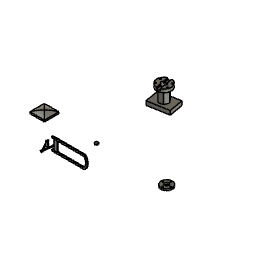
HW 1 (Autodesk Fusion 360 design; units mm, degrees)
Autodesk Fusion 360 part; units mm, degrees
note: some values were not read from the file. Set by a fixed rule: which sketch regions a step uses.
(part 1 of 2)
sketch "Sketch1" plane through (0, 0, 0) normal (0, 0, 1) x (1, 0, 0)
  line L0 (40, 0) -> (-50, 0)
  line L1 (-50, 0) -> (-50, 10)
  line L2 (-50, 10) -> (40, 10)
  line L3 (40, 10) -> (40, 0)
  line L4 (-5, 10) -> (-5, 20)
  arc A0 (40, 10) -> (-50, 10) centre (-5, -86.2) ccw
  point P0 (-5, 10)
  dimension "d1" = 10
  dimension "d2" = 90
  constraint horizontal L0
  constraint vertical L1
  constraint horizontal L2
  constraint vertical L3
  constraint midpoint L2 P0
  constraint coincident P0 L4.start
  constraint perpendicular L2 L4
  measures "d1" distance of L0.start L2.end
  measures "d2" distance of L1.end L2.end
extrude "Extrude1" add sketch "Sketch1" along normal blind 90 makes body 1
ref_plane "WorkPlane2" through (40, 5, 45) normal (1, 0, 0) x (0, 1, 0)
sketch "Sketch4" plane through (40, 5, 45) normal (1, 0, 0) x (0, 1, 0)
  line L0 (-5, 45) -> (5, 45)
  line L1 (5, 45) -> (5, -45)
  line L2 (5, -45) -> (-5, -45)
  line L3 (-5, -45) -> (-5, 45)
  line L4 (5, 0) -> (15, 0)
  arc A0 (5, -45) -> (5, 45) centre (-91.25, 0) ccw
  constraint horizontal L0
  constraint vertical L1
  constraint horizontal L2
  constraint vertical L3
  constraint midpoint L1 L4.start
  constraint perpendicular L1 L4
  constraint coincident L4.end A0
extrude "Extrude3" cut sketch "Sketch4" against normal up to surface (90 mm away) keep common part bodies 1
sketch "Sketch5" plane through (0, 0, 0) normal (0, 1, 0) x (1, 0, 0)
  circle A0 centre (220, -140) radius 35
  circle A1 centre (220, -140) radius 14
  circle A2 centre (220, -140) radius 16.5
  circle A3 centre (220, -140) radius 21
  dimension "d19" = 70
  dimension "d20" = 28
  dimension "d21" = 33
  dimension "d22" = 42
  constraint concentric A0 A1
  constraint concentric A0 A2
  constraint concentric A0 A3
  measures "d19" diameter of A0
  measures "d20" diameter of A1
  measures "d21" diameter of A2
  measures "d22" diameter of A3
extrude "Extrude4" add sketch "Sketch5" along normal blind 10 separate body contours A0 makes body 2
extrude "Extrude5" add sketch "Sketch5" along normal blind 15 contours A3 bodies 2
extrude "Extrude6" add sketch "Sketch5" along normal blind 10 contours A2 bodies 2
sketch "Sketch6" plane through (0, 10, 0) normal (0, 1, 0) x (-1, 0, 0)
  circle A0 centre (-220, 140) radius 21
  circle A1 centre (-220, 140) radius 35
ref_plane "WorkPlane3" through (220, 10, 140) normal (0, 1, 0) x (-1, 0, 0)
sketch "Sketch7" plane through (220, 10, 140) normal (0, 1, 0) x (1, 0, 0)
  circle A0 centre (0, 0) radius 25 construction
  line L0 (0, 25) -> (0, -25)
  circle A1 centre (0, -25) radius 4
  circle A2 centre (25, 0) radius 4
  circle A3 centre (0, 25) radius 4
  circle A4 centre (-25, 0) radius 4
  dimension "d30" = 50
  dimension "d31" = 8
  dimension "d33" = 360
  constraint coincident A0.centre origin
  constraint coincident A0 L0.start
  constraint coincident A0 L0.end
  constraint vertical L0
  constraint coincident L0.end A1.centre
  measures "d30" diameter of A0
  measures "d31" diameter of A1
sketch "Sketch8" plane through (220, 10, 140) normal (0, 1, 0) x (-1, 0, 0)
extrude "Extrude7" cut sketch "Sketch7" against normal up to surface (10 mm away) bodies 2
sketch "Sketch9" plane through (0, 0, 0) normal (0, 1, 0) x (1, 0, 0)
ref_plane "WorkPlane4" through (302.5, 0, -250) normal (0, -1, 0) x (1, 0, 0)
sketch "Sketch10" plane through (300, 0, -250) normal (0, -1, 0) x (1, 0, 0)
ref_plane "WorkPlane5" through (200.7071, 0, -200) normal (0, -1, 0) x (1, 0, 0)
sketch "Sketch11" plane through (230.8314, 0, -200) normal (0, -1, 0) x (1, 0, 0)
ref_plane "WorkPlane6" through (200.7071, 0, -200) normal (0, -1, 0) x (1, 0, 0)
sketch "Sketch12" plane through (243.54, 0, -200) normal (0, -1, 0) x (1, 0, 0)
sketch "Sketch13" plane through (0, 0, 0) normal (0, 1, 0) x (1, 0, 0)
  line L0 (241.0962, 97.5272) -> (441.0962, 97.5272)
  line L1 (441.0962, 157.5272) -> (241.0962, 157.5272)
  line L2 (241.0962, 157.5272) -> (241.0962, 97.5272) construction
  arc A0 (441.0962, 97.5272) -> (441.0962, 157.5272) centre (407.3666, 127.5272) ccw
  line L3 (241.0962, 87.5272) -> (445.3205, 87.5272)
  arc A1 (445.3205, 87.5272) -> (445.3205, 167.5272) centre (407.3666, 127.5272) ccw
  line L4 (445.3205, 167.5272) -> (241.0962, 167.5272)
  line L5 (241.0962, 87.5272) -> (241.0962, 97.5272)
  line L6 (241.0962, 157.5272) -> (241.0962, 167.5272)
  dimension "d124" = 200
  dimension "d134" = 60
  dimension "d136" = 10
  constraint horizontal L0
  constraint parallel L0 L1
  constraint perpendicular L0 L2
  constraint vertical L0.end L1.start
  constraint perpendicular L0 L5
  measures "d124" distance of L0.start L0.end
  measures "d134" distance of L0 L1
extrude "Extrude8" add sketch "Sketch13" along normal blind 5 separate body makes body 3
sketch "Sketch14" plane through (0, 0, 0) normal (0, 1, 0) x (1, 0, 0)
  line L0 (196.8806, 99.5126) -> (196.8806, 159.5712) construction
  line L1 (441.0962, 97.5272) -> (241.0962, 97.5272)
  point P0 (441.0962, 97.5272)
  point P1 (241.0962, 97.5272)
  point P2 (441.0962, 157.5272)
  point P3 (241.0962, 157.5272)
  constraint vertical L0
sketch "Sketch15" plane through (0, 0, 0) normal (0, 1, 0) x (1, 0, 0)
copy_body "Body->Comp2" bodies 3 removing the originals makes body 4 in component "Component"
sketch "Sketch16" plane through (0, 6.3954, 0) normal (0, 1, 0) x (-1, 0, 0)
  line L0 (-239.626, -118.3518) -> (-439.626, -118.3518)
  line L1 (-439.626, -58.3518) -> (-239.626, -58.3518)
  line L2 (-239.626, -58.3518) -> (-239.626, -118.3518) construction
  line L3 (-239.626, -48.3518) -> (-443.8504, -48.3518)
  arc A0 (-443.8504, -48.3518) -> (-443.8504, -128.3518) centre (-405.8964, -88.3518) ccw
  line L4 (-443.8504, -128.3518) -> (-239.626, -128.3518)
  line L5 (-239.626, -128.3518) -> (-239.626, -118.3518)
  arc A1 (-439.626, -58.3518) -> (-439.626, -118.3518) centre (-405.8964, -88.3518) ccw
  line L6 (-239.626, -58.3518) -> (-239.626, -48.3518)
  constraint coincident L1.end L2.start
  constraint coincident L0.start L2.end
sketch "Sketch17" plane through (0, 0, 0) normal (0, 1, 0) x (1, 0, 0)
  line L0 (146.844, 50) -> (126.844, 50)
  line L1 (126.844, 110) -> (146.844, 110)
  line L2 (146.844, 110) -> (146.844, 50)
  line L3 (239.626, 58.3518) -> (239.626, 118.3518)
  arc A0 (126.844, 90) -> (126.844, 80) centre (126.844, 85) ccw
  arc A1 (126.844, 80) -> (126.844, 90) centre (126.844, 85) ccw construction
  line L4 (126.844, 50) -> (126.844, 80)
  line L5 (126.844, 90) -> (126.844, 110)
  line L6 (126.844, 80) -> (126.844, 90) construction
  circle A2 centre (126.844, 85) radius 2.5
  dimension "d62" = 20
  dimension "d69" = 10
  dimension "d74" = 5
  constraint horizontal L0
  constraint vertical L4
  constraint horizontal L1
  constraint vertical L2
  constraint equal L2 L3
  constraint coincident A0.start L4
  constraint concentric A0 A1
  constraint coincident A0.centre L4
  constraint concentric A0 A2
  measures "d62" distance of L0.start L0.end
  measures "d69" diameter of A0
  measures "d74" diameter of A2
extrude "Extrude12" add sketch "Sketch17" along normal blind 5 separate body makes body 5
sketch "Sketch18" plane through (0, 0, 0) normal (0, 1, 0) x (1, 0, 0)
  line L0 (65, 78) -> (-50, 78)
  line L1 (-50, 78) -> (-50, 83)
  line L2 (-50, 83) -> (65, 83)
  line L3 (65, 83) -> (65, 78)
  circle A0 centre (65, 80.5) radius 5
  circle A1 centre (65, 80.5) radius 2.5
  line L4 (7.5, 78) -> (7.5, 83) construction
  circle A2 centre (-50, 80.5) radius 5
  circle A3 centre (-50, 80.5) radius 2.5
  dimension "d79" = 115
  dimension "d80" = 5
  dimension "d81" = 5
  dimension "d82" = 10
  constraint horizontal L0
  constraint vertical L1
  constraint horizontal L2
  constraint vertical L3
  constraint midpoint L3 A0.centre
  constraint concentric A0 A1
  constraint midpoint L0 L4.start
  constraint midpoint L2 L4.end
  constraint symmetric A0 L4 A2
  constraint symmetric A1 L4 A3
  measures "d79" distance of L0.start L0.end
  measures "d80" distance of L0.start L2.end
  measures "d81" diameter of A1
  measures "d82" diameter of A0
extrude "Extrude13" add sketch "Sketch18" along normal blind 5 separate body contours L0 L2 A0 A1 | L0 L2 A0 A1 | L0 L2 A0 A2 | L0 L2 A2 A3 | L0 L2 A2 A3 makes body 6
copy_body "Body->Comp3" bodies 5 removing the originals makes body 7 in component "Component'"
copy_body "Body->Comp4" bodies 6 removing the originals makes body 8 in component "Component''"
sketch "Sketch19" plane through (0, 0, 0) normal (0, 1, 0) x (1, 0, 0)
  circle A0 centre (-15, 80.5) radius 2.5
  circle A1 centre (65, 80.5) radius 2.5
  line L0 (65, 78) -> (-15, 78)
  line L1 (-15, 83) -> (65, 83)
  line L2 (-15, 78) -> (-15, 83)
  circle A2 centre (65, 80.5) radius 5
  circle A3 centre (-15, 80.5) radius 5
  line L3 (65, 83) -> (65, 78)
  line L4 (25, 78) -> (25, 83) construction
  dimension "d87" = 80
  dimension "d88" = 5
  dimension "d89" = 5
  dimension "d90" = 10
  constraint horizontal L0
  constraint vertical L2
  constraint horizontal L1
  constraint vertical L3
  constraint midpoint A1.centre L3
  constraint concentric A1 A2
  constraint midpoint L4.start L0
  constraint midpoint L4.end L1
  constraint symmetric A2 A3 L4
  constraint symmetric A0 A1 L4
  measures "d87" distance of L0.start L0.end
  measures "d88" distance of L0.start L1.end
  measures "d89" diameter of A1
  measures "d90" diameter of A2
extrude "Extrude14" add sketch "Sketch19" along normal blind 5 separate body contours A0 L0 L1 A3 | A0 L0 L1 A3 | L0 L1 A2 A3 | A1 L0 L1 A2 | A1 L0 L1 A2 makes body 9
copy_body "Body->Comp5" bodies 9 removing the originals makes body 10 in component "Component'''"
sketch "Sketch20" plane through (0, 0, 0) normal (0, 1, 0) x (1, 0, 0)
sketch "Sketch21" plane through (0, 0, 0) normal (0, 1, 0) x (1, 0, 0)
  line L0 (17.0546, 96.6667) -> (13.2961, 66.0573)
  arc A0 (8.3333, 61.6667) -> (13.2961, 66.0573) centre (8.3333, 66.6667) ccw
  line L1 (17.0546, 96.6667) -> (8.3333, 96.6667)
  line L2 (8.3333, 61.6667) -> (8.3333, 96.6667) construction
  arc A1 (3.3706, 66.0573) -> (8.3333, 61.6667) centre (8.3333, 66.6667) ccw
  line L3 (-0.388, 96.6667) -> (3.3706, 66.0573)
  line L4 (-0.388, 96.6667) -> (8.3333, 96.6667)
  circle A2 centre (8.3333, 66.6667) radius 2.5
  dimension "d97" = 5
  dimension "d98" = 5
  dimension "d157" = 30
  constraint tangent L0 A0
  constraint horizontal L1
  constraint perpendicular L1 L2
  constraint symmetric L0.start L2 L3.start
  constraint symmetric L0.end L2 A1.start
  constraint symmetric A0.start L2 A1.end
  constraint symmetric A0 L2 A1
  constraint symmetric L1.end L2 L4.end
  constraint tangent A0 A1
  constraint concentric A1 A2
  measures "d97" radius of A0
  measures "d98" diameter of A2
  measures "d157" distance of A0.centre L4
extrude "Extrude15" add sketch "Sketch21" along normal blind 5 separate body makes body 11
copy_body "Body->Comp6" bodies 11 removing the originals makes body 12 in component "Component''''"
ref_plane "WorkPlane7" through (224.2835, 10.1092, -150.504) normal (0, 0, -1) x (-1, 0, 0)
sketch "Sketch22" plane through (177.4029, 10.1092, -150.504) normal (0, 0, -1) x (1, 0, 0)
ref_plane "WorkPlane8" through (224.2835, 10.1092, -150.504) normal (0, 0, -1) x (-1, 0, 0)
copy_body "Body->Comp1" bodies 12 removing the originals makes body 13 in component "Component'''''"
sketch "Sketch24" plane through (0, 0, 0) normal (0, 0, 1) x (1, 0, 0)
sketch "Sketch25" plane through (177.4029, 10.1092, -150.504) normal (0, 0, -1) x (1, 0, 0)
sketch "Sketch26" plane through (0, 0, 0) normal (0, 0, 1) x (1, 0, 0)
move_body "Move1" bodies 1 to x (1, 0, 0) y (0, 1, 0) z (0, 0, 1) at (0, 0, 300)
move_body "Move2" bodies 2 to x (1, 0, 0) y (0, 1, 0) z (0, 0, 1) at (121.383, 0, 150)
sketch "Sketch27" plane through (0, 0, 0) normal (0, 1, 0) x (1, 0, 0)
sketch "Sketch28" plane through (0, 0, 0) normal (0, 1, 0) x (1, 0, 0)
sketch "Sketch32" plane through (0, 0, 0) normal (0, 1, 0) x (-1, 0, 0)
  line L0 (-80.1552, 73.3002) -> (-282.4188, 45.0684)
  arc A0 (-282.4188, 45.0684) -> (-271.3596, -34.1635) centre (-239.2997, 10.6992) ccw
  line L1 (-271.3596, -34.1635) -> (-69.0961, -5.9317)
  line L2 (-69.0961, -5.9317) -> (-70.4785, 3.9723)
  line L3 (-70.4785, 3.9723) -> (-268.5583, -23.6756)
  arc A1 (-276.8526, 35.7484) -> (-268.5583, -23.6756) centre (-239.2997, 10.6992) ccw
  line L4 (-276.8526, 35.7484) -> (-78.7728, 63.3962)
  line L5 (-78.7728, 63.3962) -> (-80.1552, 73.3002)
ref_plane "WorkPlane10" through (184.1141, 0, 19.5683) normal (0, 1, 0) x (-1, 0, 0)
sketch "Sketch33" plane through (184.1141, 0, 19.5683) normal (0, 1, 0) x (1, 0, 0)
  point P0 (-130, -10)
ref_plane "WorkPlane15" through (-263.0105, 97.4067, 68.3337) normal (0, -1, 0) x (-0.831247, 0, 0.555903)
sketch "Sketch36" plane through (25.171, 97.4067, 13.1125) normal (0, -1, 0) x (1, 0, 0)
ref_plane "WorkPlane17" through (-263.0105, 102.4067, 68.3337) normal (0, 1, 0) x (0.831247, 0, -0.555903)
ref_plane "WorkPlane18" through (-397.3564, 69.7422, -19.2723) normal (0, -1, 0) x (-0.831247, 0, 0.555903)
sketch "Sketch38" plane through (-397.3564, 69.7422, -19.2723) normal (0, -1, 0) x (1, 0, 0)
sketch "Sketch39" plane through (0, 0, 0) normal (0, 1, 0) x (1, 0, 0)
sketch "Sketch40" plane through (0, 0, 0) normal (0, 1, 0) x (1, 0, 0)
  line L0 (-142.9618, -165) -> (-197.629, -165)
  line L1 (-142.9618, -150) -> (-197.629, -150)
  arc A0 (-197.629, -150) -> (-197.629, -165) centre (-184.6386, -157.5) ccw
  line L2 (-142.9618, -168) -> (-199.2588, -168)
  arc A1 (-199.2588, -147) -> (-199.2588, -168) centre (-184.6386, -157.5) ccw
  line L3 (-142.9618, -147) -> (-199.2588, -147)
  line L4 (-142.9618, -168) -> (-142.9618, -165)
  line L5 (-142.9618, -150) -> (-142.9618, -147)
  dimension "d191" = 15
  dimension "d192" = 15
  dimension "d193" = 3
  constraint horizontal L0
  constraint parallel L0 L1
  constraint equal L0 L1
  constraint vertical L0.end L1.end
  constraint perpendicular L0 L4
  measures "d191" radius of A0
  measures "d192" distance of L0 L1
move_face "MoveFace1" to x (-1, 0, 0) y (0, 1, 0) z (0, 0, -1) at (850.9504, 0, -315.0544) 1 faces at (375.8376, 0, -90.8605) on bodies 4 in component "Component"
move_body "Move3" bodies 1 to x (1, 0, 0) y (0, 1, 0) z (0, 0, 1) at (-278.0793, 0, 4.8362)
move_body "Move4" bodies 2 to x (1, 0, 0) y (0, 1, 0) z (0, 0, 1) at (-152.3391, 0, 72.5424)
sketch "Sketch41" plane through (0, 0, 0) normal (0, 1, 0) x (1, 0, 0)
sketch "Sketch42" plane through (0, 0, 0) normal (0, 1, 0) x (1, 0, 0)
  spline S0 degree 5 poles (330, -40) (329.982, -39.3508) (329.8566, -38.0719) (329.3466, -36.2401) (327.9023, -34.0517) (324.8647, -31.8237) (320.8722, -30.1154) (316.3282, -28.9135) (311.6472, -28.2306) (307.2063, -28.101) (303.3111, -28.5644) (300.1557, -29.6535) (297.7883, -31.3809) (296.0647, -33.7246) (294.7251, -36.6338) (293.4885, -40.0382) (292.1424, -43.8558) (290.6295, -48.0012) (288.9995, -52.3891) (287.3657, -56.9385) (285.8583, -61.5763) (284.5828, -66.2408) (283.567, -70.8865) (282.7481, -75.4848) (282.0163, -80.0212) (281.2434, -84.4931) (280.319, -88.907) (279.1806, -93.2764) (277.8542, -97.6192) (276.4355, -101.9555) (275.0528, -106.3057) (273.8348, -110.6882) (272.8782, -115.1177) (272.2117, -119.603) (271.7717, -124.1447) (271.4365, -128.7327) (271.0527, -133.3436) (270.4666, -137.9376) (269.5496, -142.4568) (268.234, -146.8204) (266.5133, -150.932) (264.4142, -154.6981) (261.9746, -158.0441) (259.2224, -160.9292) (256.1482, -163.3664) (252.6982, -165.4256) (248.8192, -167.1956) (244.4931, -168.7534) (239.775, -170.131) (234.8317, -171.2827) (229.9745, -172.0554) (225.5771, -172.2416) (221.9992, -171.6295) (219.509, -170.0518) (218.2022, -167.4389) (217.9357, -163.8616) (218.4166, -159.4871) (219.28, -154.5411) (220.1687, -149.2682) (220.8165, -143.8915) (221.1164, -138.578) (221.0744, -133.4453) (220.7773, -128.5641) (220.3549, -123.9626) (219.9446, -119.6293) (219.6541, -115.5171) (219.5282, -111.5472) (219.5676, -107.6249) (219.7444, -103.6547) (220.0192, -99.5557) (220.357, -95.277) (220.743, -90.8116) (221.1746, -86.1889) (221.6572, -81.4698) (222.1981, -76.7408) (222.8017, -72.1077) (223.4629, -67.6925) (224.165, -63.6149) (224.881, -59.9585) (225.5732, -56.7376) (226.1955, -53.8724) (226.6895, -51.1395) (227.0099, -48.2472) (227.162, -44.9651) (227.2347, -41.2351) (227.4373, -37.2945) (228.0296, -33.5588) (229.2449, -30.4954) (231.2234, -28.5099) (233.9229, -27.8017) (237.1375, -28.3709) (240.5673, -30.0963) (243.8732, -32.7935) (246.7341, -36.2739) (248.8725, -40.3478) (250.0855, -44.8364) (250.2738, -49.5801) (249.4703, -54.4478) (247.8733, -59.3474) (245.7928, -64.2212) (243.5888, -69.0414) (241.614, -73.8053) (240.1513, -78.5308) (239.3609, -83.2512) (239.2048, -88.0114) (239.4831, -92.8569) (239.9203, -97.8186) (240.2331, -102.899) (240.211, -108.0576) (239.7799, -113.1986) (239.1014, -118.151) (238.5246, -122.6855) (238.4551, -126.5533) (239.2423, -129.5202) (241.074, -131.3989) (243.8313, -132.0894) (247.1479, -131.5816) (250.5689, -129.9395) (253.6856, -127.2913) (256.2572, -123.8157) (258.1708, -119.7171) (259.4204, -115.2018) (260.0786, -110.4537) (260.2721, -105.6106) (260.1547, -100.7384) (259.893, -95.8485) (259.6537, -90.9204) (259.5902, -85.9223) (259.8289, -80.8324) (260.4572, -75.659) (261.5075, -70.4651) (262.9644, -65.3503) (264.7744, -60.4244) (266.8549, -55.785) (269.1032, -51.4913) (271.4066, -47.5439) (273.6498, -43.8516) (275.7303, -40.2533) (277.5751, -36.5733) (279.1598, -32.6694) (280.5228, -28.4781) (281.7892, -24.0742) (283.1662, -19.6799) (284.8918, -15.5878) (287.1921, -12.1014) (290.2379, -9.4708) (294.0974, -7.826) (298.7, -7.1244) (303.8774, -7.2117) (309.3962, -7.8713) (314.9942, -8.8786) (320.4151, -10.0519) (325.4443, -11.3073) (329.9419, -12.7057) (333.8308, -14.3914) (337.0863, -16.5356) (339.7255, -19.2768) (341.7966, -22.6665) (343.3695, -26.6012) (344.512, -30.8609) (345.2645, -35.1694) (345.6119, -39.2484) (345.4641, -42.8698) (344.6124, -45.9216) (342.845, -48.3723) (340.1079, -50.204) (336.6505, -51.3567) (333.1761, -51.6684) (330.4812, -50.9811) (329.1531, -49.228) (329.1476, -46.5586) (329.6685, -43.9727) (329.9643, -41.9668) (330.018, -40.6492) (330, -40) knots 0 0 0 0 0 0 0.00588235 0.01176471 0.01764706 0.02352941 0.02941176 0.03529412 0.04117647 0.04705882 0.05294118 0.05882353 0.06470588 0.07058824 0.07647059 0.08235294 0.08823529 0.09411765 0.1 0.10588235 0.11176471 0.11764706 0.12352941 0.12941176 0.13529412 0.14117647 0.14705882 0.15294118 0.15882353 0.16470588 0.17058824 0.17647059 0.18235294 0.18823529 0.19411765 0.2 0.20588235 0.21176471 0.21764706 0.22352941 0.22941176 0.23529412 0.24117647 0.24705882 0.25294118 0.25882353 0.26470588 0.27058824 0.27647059 0.28235294 0.28823529 0.29411765 0.3 0.30588235 0.31176471 0.31764706 0.32352941 0.32941176 0.33529412 0.34117647 0.34705882 0.35294118 0.35882353 0.36470588 0.37058824 0.37647059 0.38235294 0.38823529 0.39411765 0.4 0.40588235 0.41176471 0.41764706 0.42352941 0.42941176 0.43529412 0.44117647 0.44705882 0.45294118 0.45882353 0.46470588 0.47058824 0.47647059 0.48235294 0.48823529 0.49411765 0.5 0.50588235 0.51176471 0.51764706 0.52352941 0.52941176 0.53529412 0.54117647 0.54705882 0.55294118 0.55882353 0.56470588 0.57058824 0.57647059 0.58235294 0.58823529 0.59411765 0.6 0.60588235 0.61176471 0.61764706 0.62352941 0.62941176 0.63529412 0.64117647 0.64705882 0.65294118 0.65882353 0.66470588 0.67058824 0.67647059 0.68235294 0.68823529 0.69411765 0.7 0.70588235 0.71176471 0.71764706 0.72352941 0.72941176 0.73529412 0.74117647 0.74705882 0.75294118 0.75882353 0.76470588 0.77058824 0.77647059 0.78235294 0.78823529 0.79411765 0.8 0.80588235 0.81176471 0.81764706 0.82352941 0.82941176 0.83529412 0.84117647 0.84705882 0.85294118 0.85882353 0.86470588 0.87058824 0.87647059 0.88235294 0.88823529 0.89411765 0.9 0.90588235 0.91176471 0.91764706 0.92352941 0.92941176 0.93529412 0.94117647 0.94705882 0.95294118 0.95882353 0.96470588 0.97058824 0.97647059 0.98235294 0.98823529 0.99411765 1 1 1 1 1 1
  spline S1 degree 5 poles (200, -70) (199.8209, -70.5454) (199.4785, -71.6619) (199.0137, -73.4203) (198.4826, -75.9426) (197.8855, -79.3596) (197.2368, -82.9658) (196.403, -86.6581) (195.2576, -90.3207) (193.7011, -93.8392) (191.6868, -97.1173) (189.2302, -100.0861) (186.3917, -102.6988) (183.2646, -104.9292) (179.9612, -106.7679) (176.5995, -108.2204) (173.2904, -109.3036) (170.1223, -110.044) (167.1547, -110.4718) (164.421, -110.6097) (161.9296, -110.4633) (159.6661, -110.011) (157.5944, -109.1923) (155.6594, -107.9026) (153.7997, -106.0333) (151.9595, -103.5073) (150.1011, -100.3168) (148.2162, -96.5589) (146.339, -92.4756) (144.5339, -88.4062) (142.882, -84.7365) (141.4678, -81.8493) (140.3661, -80.0723) (139.6288, -79.6322) (139.2707, -80.5948) (139.2632, -82.8523) (139.5436, -86.1728) (140.0193, -90.2344) (140.5744, -94.6652) (141.0755, -99.0804) (141.3886, -103.1135) (141.3951, -106.4483) (141.0073, -108.8491) (140.1853, -110.1938) (138.9521, -110.5024) (137.4119, -109.9755) (135.7171, -108.8865) (134.0309, -107.4619) (132.4913, -105.7662) (131.2054, -103.7623) (130.243, -101.3752) (129.6322, -98.5496) (129.3509, -95.3231) (129.3328, -91.834) (129.4876, -88.2687) (129.7162, -84.8263) (129.9293, -81.6753) (130.0621, -78.9174) (130.0956, -76.5375) (130.0594, -74.3974) (130.0048, -72.3014) (129.9844, -70.0467) (130.0285, -67.4795) (130.1242, -64.5482) (130.23, -61.281) (130.2904, -57.764) (130.2511, -54.119) (130.0738, -50.4819) (129.7502, -46.9806) (129.3197, -43.7118) (128.8485, -40.7373) (128.4025, -38.0837) (128.0211, -35.7402) (127.6945, -33.6596) (127.3292, -31.7519) (126.7557, -29.9019) (125.8014, -28.0258) (124.3406, -26.1109) (122.37, -24.28) (120.0098, -22.7717) (117.4423, -21.847) (114.8665, -21.7134) (112.449, -22.4493) (110.2686, -23.9084) (108.3263, -25.7775) (106.5739, -27.6748) (104.9361, -29.2333) (103.3353, -30.1942) (101.7162, -30.4856) (100.0813, -30.16) (98.5241, -29.3424) (97.2695, -28.173) (96.5709, -26.7766) (96.6007, -25.2348) (97.336, -23.5526) (98.6256, -21.7002) (100.2657, -19.6554) (102.0786, -17.4501) (103.9728, -15.2021) (105.9142, -13.0743) (107.9081, -11.2429) (109.9777, -9.8624) (112.1433, -9.0322) (114.4023, -8.7621) (116.7368, -8.9957) (119.1237, -9.6334) (121.5416, -10.5554) (123.9825, -11.6464) (126.4464, -12.8076) (128.927, -13.9618) (131.3997, -15.0607) (133.8106, -16.0899) (136.0591, -17.078) (138.0102, -18.0928) (139.5337, -19.2299) (140.5328, -20.6006) (140.9834, -22.3252) (140.945, -24.507) (140.5392, -27.1828) (139.9372, -30.2821) (139.3441, -33.577) (138.9818, -36.6515) (139.0413, -39.0239) (139.6351, -40.2615) (140.756, -40.0882) (142.2158, -38.5221) (143.7067, -35.828) (144.9018, -32.4116) (145.5475, -28.7288) (145.5479, -25.1964) (145.0825, -22.0837) (144.5497, -19.5075) (144.4256, -17.4778) (145.1484, -15.9269) (146.9934, -14.7459) (149.9487, -13.8179) (153.7876, -13.0315) (158.1489, -12.2925) (162.6132, -11.5363) (166.7817, -10.7405) (170.3526, -9.9363) (173.2016, -9.2224) (175.4523, -8.7739) (177.3748, -8.7927) (179.2879, -9.4565) (181.4677, -10.8743) (184.0345, -13.0262) (186.9556, -15.7777) (190.097, -18.9248) (193.261, -22.2296) (196.2282, -25.459) (198.7993, -28.4241) (200.8332, -31.0145) (202.2964, -33.2464) (203.273, -35.2655) (203.9052, -37.2742) (204.3481, -39.4739) (204.7224, -42.0056) (205.0592, -44.8799) (205.3183, -48.0037) (205.4228, -51.2285) (205.2884, -54.3909) (204.8533, -57.3555) (204.1111, -60.0603) (203.1336, -62.5492) (202.0345, -64.931) (201.159, -66.8634) (200.5529, -68.3897) (200.1791, -69.4546) (200, -70) knots 0 0 0 0 0 0 0.00606061 0.01212121 0.01818182 0.02424242 0.03030303 0.03636364 0.04242424 0.04848485 0.05454545 0.06060606 0.06666667 0.07272727 0.07878788 0.08484848 0.09090909 0.0969697 0.1030303 0.10909091 0.11515152 0.12121212 0.12727273 0.13333333 0.13939394 0.14545455 0.15151515 0.15757576 0.16363636 0.16969697 0.17575758 0.18181818 0.18787879 0.19393939 0.2 0.20606061 0.21212121 0.21818182 0.22424242 0.23030303 0.23636364 0.24242424 0.24848485 0.25454545 0.26060606 0.26666667 0.27272727 0.27878788 0.28484848 0.29090909 0.2969697 0.3030303 0.30909091 0.31515152 0.32121212 0.32727273 0.33333333 0.33939394 0.34545455 0.35151515 0.35757576 0.36363636 0.36969697 0.37575758 0.38181818 0.38787879 0.39393939 0.4 0.40606061 0.41212121 0.41818182 0.42424242 0.43030303 0.43636364 0.44242424 0.44848485 0.45454545 0.46060606 0.46666667 0.47272727 0.47878788 0.48484848 0.49090909 0.4969697 0.5030303 0.50909091 0.51515152 0.52121212 0.52727273 0.53333333 0.53939394 0.54545455 0.55151515 0.55757576 0.56363636 0.56969697 0.57575758 0.58181818 0.58787879 0.59393939 0.6 0.60606061 0.61212121 0.61818182 0.62424242 0.63030303 0.63636364 0.64242424 0.64848485 0.65454545 0.66060606 0.66666667 0.67272727 0.67878788 0.68484848 0.69090909 0.6969697 0.7030303 0.70909091 0.71515152 0.72121212 0.72727273 0.73333333 0.73939394 0.74545455 0.75151515 0.75757576 0.76363636 0.76969697 0.77575758 0.78181818 0.78787879 0.79393939 0.8 0.80606061 0.81212121 0.81818182 0.82424242 0.83030303 0.83636364 0.84242424 0.84848485 0.85454545 0.86060606 0.86666667 0.87272727 0.87878788 0.88484848 0.89090909 0.8969697 0.9030303 0.90909091 0.91515152 0.92121212 0.92727273 0.93333333 0.93939394 0.94545455 0.95151515 0.95757576 0.96363636 0.96969697 0.97575758 0.98181818 0.98787879 0.99393939 1 1 1 1 1 1
  spline S2 degree 5 poles (180, -70) (180.1552, -70.6341) (180.4704, -71.8781) (180.9283, -73.6534) (181.3732, -75.7944) (181.3, -78.0819) (180.3066, -80.0251) (178.2399, -81.6823) (175.1631, -83.0809) (171.3018, -84.2203) (166.987, -85.0742) (162.5997, -85.5936) (158.5154, -85.7098) (155.0477, -85.3365) (152.3953, -84.3734) (150.6535, -82.7308) (149.8209, -80.3531) (149.8083, -77.2423) (150.445, -73.4831) (151.5115, -69.2227) (152.7727, -64.6464) (154.0111, -59.9557) (155.0604, -55.3451) (155.8377, -50.9797) (156.3803, -46.971) (156.8685, -43.3594) (157.5545, -40.148) (158.7037, -37.3282) (160.5294, -34.9107) (163.1352, -32.9499) (166.4397, -31.5818) (170.211, -30.9856) (174.1301, -31.3281) (177.8464, -32.7098) (181.0328, -35.1165) (183.4482, -38.3543) (184.9758, -42.0369) (185.6011, -45.7109) (185.4023, -48.9545) (184.5351, -51.487) (183.2212, -53.2736) (181.7347, -54.6314) (180.3541, -56.0241) (179.3187, -57.8846) (178.7746, -60.3835) (178.7604, -63.4192) (179.125, -66.0814) (179.5393, -68.0737) (179.8448, -69.3659) (180, -70) knots 0 0 0 0 0 0 0.022222 0.044444 0.066667 0.088889 0.111111 0.133333 0.155556 0.177778 0.2 0.222222 0.244444 0.266667 0.288889 0.311111 0.333333 0.355556 0.377778 0.4 0.422222 0.444444 0.466667 0.488889 0.511111 0.533333 0.555556 0.577778 0.6 0.622222 0.644444 0.666667 0.688889 0.711111 0.733333 0.755556 0.777778 0.8 0.822222 0.844444 0.866667 0.888889 0.911111 0.933333 0.955556 0.977778 1 1 1 1 1 1
  spline S3 degree 5 poles (54.6306, -110.3194) (54.531, -109.7401) (54.3312, -108.5102) (54.0541, -106.4282) (53.8004, -103.1409) (53.7506, -98.2975) (53.9614, -92.9794) (54.3669, -87.5185) (54.8642, -82.2469) (55.3345, -77.4324) (55.6667, -73.1948) (55.7722, -69.496) (55.5908, -66.1987) (55.101, -63.1064) (54.3257, -60.0088) (53.3448, -56.7314) (52.2873, -53.1609) (51.295, -49.238) (50.4936, -44.9585) (49.9607, -40.3705) (49.6961, -35.5736) (49.5876, -30.7177) (49.4441, -25.9819) (49.0333, -21.551) (48.1165, -17.5932) (46.4863, -14.2367) (44.0008, -11.5484) (40.6236, -9.5082) (36.4084, -8.0328) (31.4814, -7.0037) (26.0234, -6.2933) (20.252, -5.7926) (14.4045, -5.4358) (8.7199, -5.2333) (3.4222, -5.275) (-1.2942, -5.6924) (-5.279, -6.6316) (-8.4419, -8.2202) (-10.7658, -10.5397) (-12.3255, -13.59) (-13.2898, -17.2739) (-13.8762, -21.4358) (-14.3154, -25.8891) (-14.8103, -30.4498) (-15.5009, -34.9642) (-16.4176, -39.346) (-17.496, -43.5735) (-18.6146, -47.6742) (-19.6244, -51.7136) (-20.3825, -55.7822) (-20.7821, -59.983) (-20.7899, -64.4192) (-20.4397, -69.1782) (-19.8129, -74.3124) (-19.0235, -79.8215) (-18.2011, -85.6355) (-17.4746, -91.5941) (-16.9564, -97.4342) (-16.7237, -102.7583) (-16.814, -107.0781) (-17.2318, -109.9138) (-17.9528, -110.8817) (-18.9286, -109.7792) (-20.091, -106.6882) (-21.3583, -101.9252) (-22.6414, -95.9582) (-23.8502, -89.3344) (-24.8994, -82.6053) (-25.7153, -76.2495) (-26.2416, -70.6036) (-26.446, -65.7709) (-26.3242, -61.6559) (-25.9039, -58.0437) (-25.2478, -54.6653) (-24.4574, -51.2682) (-23.6766, -47.6855) (-23.0952, -43.9045) (-22.9028, -40.0174) (-23.2442, -36.1737) (-24.172, -32.5309) (-25.6054, -29.2083) (-27.2732, -26.2326) (-28.8109, -23.5537) (-29.889, -21.0694) (-30.3155, -18.6483) (-30.1857, -16.1503) (-29.8557, -13.4616) (-29.7754, -10.5446) (-30.368, -7.4772) (-31.8757, -4.5112) (-34.3501, -1.996) (-37.6617, -0.2727) (-41.5103, 0.4116) (-45.4195, 0.0216) (-48.7924, -1.2462) (-51.0733, -3.0984) (-51.8727, -5.2352) (-51.1318, -7.4736) (-49.1936, -9.8124) (-46.6029, -12.3414) (-43.9554, -15.1784) (-41.7225, -18.393) (-40.1009, -21.9427) (-39.0936, -25.7162) (-38.5777, -29.5702) (-38.3776, -33.3694) (-38.3325, -37.0234) (-38.3766, -40.5304) (-38.5162, -43.9562) (-38.7884, -47.4006) (-39.2258, -50.9683) (-39.8206, -54.7386) (-40.4849, -58.7336) (-41.0822, -62.9277) (-41.4622, -67.26) (-41.4955, -71.6456) (-41.1064, -75.9869) (-40.311, -80.1858) (-39.2398, -84.1544) (-38.0748, -87.8224) (-36.9969, -91.1449) (-36.1282, -94.11) (-35.4796, -96.7467) (-34.8888, -99.1322) (-34.1309, -101.3824) (-33.0222, -103.6383) (-31.5545, -106.0599) (-29.9147, -108.7936) (-28.3491, -111.9026) (-27.0661, -115.3057) (-26.1234, -118.7148) (-25.3216, -121.568) (-24.3489, -123.3228) (-22.9077, -123.6898) (-20.8808, -123.0032) (-18.3554, -122.1029) (-15.5152, -121.7957) (-12.5572, -122.3427) (-9.6329, -123.2081) (-6.8905, -123.5807) (-4.4899, -122.6966) (-2.642, -120.3288) (-1.5901, -116.8895) (-1.517, -113.0575) (-2.4761, -109.5339) (-4.3008, -106.719) (-6.5599, -104.5056) (-8.7112, -102.5075) (-10.2276, -100.231) (-10.7335, -97.2663) (-10.1395, -93.475) (-8.5782, -88.9284) (-6.333, -83.8383) (-3.7715, -78.4914) (-1.2744, -73.1803) (0.8289, -68.1412) (2.3387, -63.4748) (3.22, -59.1231) (3.5573, -54.9501) (3.5276, -50.798) (3.3663, -46.5564) (3.3361, -42.2193) (3.6943, -37.9624) (4.6612, -34.1656) (6.392, -31.2839) (8.9455, -29.7392) (12.259, -29.8142) (16.1083, -31.5198) (20.1481, -34.6246) (23.985, -38.7495) (27.2384, -43.4396) (29.6093, -48.2481) (30.9387, -52.8087) (31.2877, -56.9286) (30.9518, -60.6222) (30.3397, -64.0269) (29.8772, -67.341) (29.9073, -70.7562) (30.5785, -74.3851) (31.7796, -78.2139) (33.2516, -82.1539) (34.6685, -86.0757) (35.7342, -89.8517) (36.2643, -93.3926) (36.2948, -96.693) (36.0278, -99.8149) (35.7361, -102.854) (35.6878, -105.9123) (36.0481, -109.0677) (36.8368, -112.3473) (37.994, -115.7115) (39.4268, -119.031) (41.0569, -122.077) (42.8856, -124.4802) (44.9577, -125.8332) (47.2785, -125.8548) (49.7388, -124.5493) (52.057, -122.3253) (53.9119, -119.7354) (55.0452, -117.2746) (55.3945, -115.1187) (55.2022, -113.4272) (54.9292, -111.9862) (54.7303, -110.8987) (54.6306, -110.3194) knots 0 0 0 0 0 0 0.005 0.01 0.015 0.02 0.025 0.03 0.035 0.04 0.045 0.05 0.055 0.06 0.065 0.07 0.075 0.08 0.085 0.09 0.095 0.1 0.105 0.11 0.115 0.12 0.125 0.13 0.135 0.14 0.145 0.15 0.155 0.16 0.165 0.17 0.175 0.18 0.185 0.19 0.195 0.2 0.205 0.21 0.215 0.22 0.225 0.23 0.235 0.24 0.245 0.25 0.255 0.26 0.265 0.27 0.275 0.28 0.285 0.29 0.295 0.3 0.305 0.31 0.315 0.32 0.325 0.33 0.335 0.34 0.345 0.35 0.355 0.36 0.365 0.37 0.375 0.38 0.385 0.39 0.395 0.4 0.405 0.41 0.415 0.42 0.425 0.43 0.435 0.44 0.445 0.45 0.455 0.46 0.465 0.47 0.475 0.48 0.485 0.49 0.495 0.5 0.505 0.51 0.515 0.52 0.525 0.53 0.535 0.54 0.545 0.55 0.555 0.56 0.565 0.57 0.575 0.58 0.585 0.59 0.595 0.6 0.605 0.61 0.615 0.62 0.625 0.63 0.635 0.64 0.645 0.65 0.655 0.66 0.665 0.67 0.675 0.68 0.685 0.69 0.695 0.7 0.705 0.71 0.715 0.72 0.725 0.73 0.735 0.74 0.745 0.75 0.755 0.76 0.765 0.77 0.775 0.78 0.785 0.79 0.795 0.8 0.805 0.81 0.815 0.82 0.825 0.83 0.835 0.84 0.845 0.85 0.855 0.86 0.865 0.87 0.875 0.88 0.885 0.89 0.895 0.9 0.905 0.91 0.915 0.92 0.925 0.93 0.935 0.94 0.945 0.95 0.955 0.96 0.965 0.97 0.975 0.98 0.985 0.99 0.995 1 1 1 1 1 1
  spline S4 degree 5 poles (34.8564, -150.3174) (35.1138, -150.4614) (35.629, -150.8107) (36.4134, -151.5265) (37.4829, -152.8752) (38.7346, -155.1489) (39.714, -157.872) (40.2331, -160.8606) (40.175, -163.9116) (39.5331, -166.8236) (38.3674, -169.4085) (36.777, -171.5043) (34.8667, -172.9874) (32.7154, -173.7856) (30.3449, -173.8907) (27.741, -173.3529) (24.8735, -172.2763) (21.7171, -170.8146) (18.2698, -169.165) (14.5773, -167.5677) (10.7357, -166.2839) (6.8715, -165.5547) (3.1287, -165.5637) (-0.3473, -166.4003) (-3.4241, -168.0173) (-5.9973, -170.2026) (-8.0076, -172.516) (-9.446, -174.349) (-10.3476, -175.1282) (-10.7864, -174.4609) (-10.8731, -172.3515) (-10.7398, -169.2141) (-10.5078, -165.6557) (-10.2598, -162.3174) (-10.01, -159.6934) (-9.6756, -157.9565) (-9.048, -156.7898) (-7.8971, -155.6568) (-6.0572, -154.0309) (-3.5449, -151.6916) (-0.566, -148.7837) (2.576, -145.6649) (5.5444, -142.8122) (8.0425, -140.7066) (9.8876, -139.7229) (11.0759, -140.0271) (11.8745, -141.4432) (12.7063, -143.5556) (13.9884, -145.8628) (15.9878, -147.9115) (18.6668, -149.4414) (21.7834, -150.3544) (24.9886, -150.684) (27.9301, -150.5655) (30.343, -150.2053) (32.1697, -149.8521) (33.3048, -149.7809) (34.0847, -149.9464) (34.599, -150.1733) (34.8564, -150.3174) knots 0 0 0 0 0 0 0.018182 0.036364 0.054545 0.072727 0.090909 0.109091 0.127273 0.145455 0.163636 0.181818 0.2 0.218182 0.236364 0.254545 0.272727 0.290909 0.309091 0.327273 0.345455 0.363636 0.381818 0.4 0.418182 0.436364 0.454545 0.472727 0.490909 0.509091 0.527273 0.545455 0.563636 0.581818 0.6 0.618182 0.636364 0.654545 0.672727 0.690909 0.709091 0.727273 0.745455 0.763636 0.781818 0.8 0.818182 0.836364 0.854545 0.872727 0.890909 0.909091 0.927273 0.945455 0.963636 0.981818 1 1 1 1 1 1
  spline S5 degree 5 poles (-70, -180) (-70.3601, -180.1728) (-71.1425, -180.437) (-72.4957, -180.6031) (-74.6121, -180.4749) (-77.5932, -180.1159) (-80.6964, -179.9081) (-83.7189, -180.0037) (-86.501, -180.2551) (-88.9298, -180.3482) (-90.9449, -179.894) (-92.5482, -178.5469) (-93.7974, -176.0749) (-94.7808, -172.3802) (-95.5959, -167.5312) (-96.3273, -161.7904) (-97.0241, -155.6444) (-97.7099, -149.7141) (-98.3941, -144.6616) (-99.0814, -141.1011) (-99.7835, -139.5032) (-100.5283, -140.1125) (-101.3729, -142.8334) (-102.3971, -147.2807) (-103.689, -152.8899) (-105.3329, -159.008) (-107.3969, -164.9926) (-109.9199, -170.3071) (-112.8995, -174.6183) (-116.2791, -177.8914) (-119.9645, -180.2991) (-123.84, -182.1331) (-127.784, -183.7157) (-131.6855, -185.3074) (-135.4594, -187.0269) (-139.0649, -188.7378) (-142.5029, -190.1253) (-145.806, -190.8274) (-149.0315, -190.5552) (-152.2523, -189.203) (-155.5508, -186.9997) (-158.9989, -184.431) (-162.6314, -182.0656) (-166.4223, -180.4109) (-170.2597, -179.7592) (-173.92, -180.0323) (-177.0477, -180.6441) (-179.3014, -180.8312) (-180.4768, -179.9354) (-180.669, -177.757) (-180.3222, -174.711) (-179.9518, -171.4243) (-179.9559, -168.4738) (-180.3275, -165.9843) (-180.6611, -163.6191) (-180.4558, -160.9621) (-179.3162, -157.7625) (-177.2488, -154.3115) (-174.591, -151.3101) (-171.8089, -149.5555) (-169.3464, -149.7007) (-167.4329, -151.9503) (-165.9711, -155.8876) (-164.6806, -160.7319) (-163.1971, -165.5225) (-161.1963, -169.3404) (-158.4921, -171.493) (-155.1828, -171.7685) (-151.6116, -170.4165) (-148.2051, -167.9466) (-145.3432, -164.9771) (-143.2266, -162.0703) (-141.7172, -159.5539) (-140.4588, -157.5382) (-139.053, -155.9713) (-137.2126, -154.6816) (-134.9338, -153.4243) (-132.396, -151.9439) (-129.8487, -150.0367) (-127.5018, -147.6151) (-125.4189, -144.7668) (-123.5559, -141.6852) (-121.7941, -138.6034) (-119.975, -135.7286) (-117.9352, -133.1722) (-115.5397, -130.8945) (-112.7155, -128.7675) (-109.4827, -126.6278) (-105.988, -124.333) (-102.5366, -121.8157) (-99.6253, -119.1408) (-97.8156, -116.4649) (-97.5938, -113.9939) (-99.252, -111.9433) (-102.7235, -110.4923) (-107.6145, -109.7638) (-113.3446, -109.8184) (-119.2539, -110.644) (-124.7249, -112.1469) (-129.2949, -114.1433) (-132.7793, -116.3487) (-135.3732, -118.3733) (-137.4748, -119.8086) (-139.5172, -120.3129) (-141.81, -119.6888) (-144.3453, -117.9838) (-146.8766, -115.4253) (-149.0653, -112.3157) (-150.5951, -108.9478) (-151.3194, -105.4958) (-151.3312, -101.9682) (-150.8716, -98.2917) (-150.2711, -94.3684) (-149.877, -90.1443) (-149.9879, -85.6719) (-150.7838, -81.1775) (-152.3409, -76.9859) (-154.6485, -73.4444) (-157.6245, -70.8437) (-161.1315, -69.3472) (-164.9927, -68.8998) (-169.0094, -69.2032) (-172.9817, -69.8299) (-176.7298, -70.3068) (-180.1141, -70.211) (-183.0565, -69.2606) (-185.5603, -67.4075) (-187.6657, -64.782) (-189.4011, -61.6375) (-190.7437, -58.2964) (-191.5581, -55.0925) (-191.6167, -52.3261) (-190.7041, -50.228) (-188.6896, -48.9253) (-185.633, -48.3959) (-181.7522, -48.4939) (-177.3467, -49.0005) (-172.7321, -49.667) (-168.1771, -50.2588) (-163.8241, -50.6052) (-159.6683, -50.6244) (-155.6276, -50.3077) (-151.5905, -49.713) (-147.476, -48.9556) (-143.2802, -48.1986) (-139.1481, -47.6464) (-135.3651, -47.5256) (-132.2495, -48.0482) (-130.067, -49.3783) (-128.9438, -51.6003) (-128.7596, -54.6787) (-129.1988, -58.479) (-129.8398, -62.8037) (-130.2351, -67.4243) (-129.9887, -72.1127) (-128.8492, -76.6784) (-126.7421, -80.9825) (-123.7229, -84.9224) (-119.9505, -88.4236) (-115.6535, -91.429) (-111.0983, -93.8892) (-106.5576, -95.7528) (-102.2758, -96.9542) (-98.4565, -97.4232) (-95.2547, -97.1009) (-92.7682, -95.9544) (-91.0301, -93.9905) (-89.9971, -91.2737) (-89.567, -87.9152) (-89.6058, -84.0537) (-89.9716, -79.8389) (-90.5397, -75.4131) (-91.2262, -70.8949) (-91.9707, -66.3835) (-92.7199, -61.9625) (-93.4124, -57.7037) (-93.9612, -53.671) (-94.2402, -49.9243) (-94.0612, -46.523) (-93.2222, -43.5328) (-91.5722, -41.0336) (-89.0634, -39.1246) (-85.826, -37.9366) (-82.1705, -37.6218) (-78.4876, -38.3149) (-75.1704, -40.0994) (-72.5334, -42.9753) (-70.7165, -46.8159) (-69.695, -51.3901) (-69.3345, -56.41) (-69.4307, -61.5701) (-69.7565, -66.5917) (-70.1036, -71.2614) (-70.3318, -75.4799) (-70.3981, -79.2843) (-70.3223, -82.7989) (-70.1647, -86.1968) (-69.9982, -89.6574) (-69.884, -93.3272) (-69.8432, -97.2749) (-69.8662, -101.5044) (-69.925, -105.9704) (-69.9839, -110.5932) (-70.0117, -115.2746) (-69.9917, -119.9123) (-69.9359, -124.4163) (-69.8753, -128.7148) (-69.8464, -132.7584) (-69.8796, -136.5249) (-69.9859, -140.0236) (-70.1452, -143.3) (-70.2931, -146.4407) (-70.346, -149.5512) (-70.2268, -152.7332) (-69.8884, -156.0638) (-69.3435, -159.5702) (-68.6726, -163.218) (-68.0001, -166.9203) (-67.478, -170.5404) (-67.267, -173.8996) (-67.5184, -176.7757) (-68.1871, -178.5) (-68.9816, -179.4) (-69.6399, -179.8272) (-70, -180) knots 0 0 0 0 0 0 0.00454545 0.00909091 0.01363636 0.01818182 0.02272727 0.02727273 0.03181818 0.03636364 0.04090909 0.04545455 0.05 0.05454545 0.05909091 0.06363636 0.06818182 0.07272727 0.07727273 0.08181818 0.08636364 0.09090909 0.09545455 0.1 0.10454545 0.10909091 0.11363636 0.11818182 0.12272727 0.12727273 0.13181818 0.13636364 0.14090909 0.14545455 0.15 0.15454545 0.15909091 0.16363636 0.16818182 0.17272727 0.17727273 0.18181818 0.18636364 0.19090909 0.19545455 0.2 0.20454545 0.20909091 0.21363636 0.21818182 0.22272727 0.22727273 0.23181818 0.23636364 0.24090909 0.24545455 0.25 0.25454545 0.25909091 0.26363636 0.26818182 0.27272727 0.27727273 0.28181818 0.28636364 0.29090909 0.29545455 0.3 0.30454545 0.30909091 0.31363636 0.31818182 0.32272727 0.32727273 0.33181818 0.33636364 0.34090909 0.34545455 0.35 0.35454545 0.35909091 0.36363636 0.36818182 0.37272727 0.37727273 0.38181818 0.38636364 0.39090909 0.39545455 0.4 0.40454545 0.40909091 0.41363636 0.41818182 0.42272727 0.42727273 0.43181818 0.43636364 0.44090909 0.44545455 0.45 0.45454545 0.45909091 0.46363636 0.46818182 0.47272727 0.47727273 0.48181818 0.48636364 0.49090909 0.49545455 0.5 0.50454545 0.50909091 0.51363636 0.51818182 0.52272727 0.52727273 0.53181818 0.53636364 0.54090909 0.54545455 0.55 0.55454545 0.55909091 0.56363636 0.56818182 0.57272727 0.57727273 0.58181818 0.58636364 0.59090909 0.59545455 0.6 0.60454545 0.60909091 0.61363636 0.61818182 0.62272727 0.62727273 0.63181818 0.63636364 0.64090909 0.64545455 0.65 0.65454545 0.65909091 0.66363636 0.66818182 0.67272727 0.67727273 0.68181818 0.68636364 0.69090909 0.69545455 0.7 0.70454545 0.70909091 0.71363636 0.71818182 0.72272727 0.72727273 0.73181818 0.73636364 0.74090909 0.74545455 0.75 0.75454545 0.75909091 0.76363636 0.76818182 0.77272727 0.77727273 0.78181818 0.78636364 0.79090909 0.79545455 0.8 0.80454545 0.80909091 0.81363636 0.81818182 0.82272727 0.82727273 0.83181818 0.83636364 0.84090909 0.84545455 0.85 0.85454545 0.85909091 0.86363636 0.86818182 0.87272727 0.87727273 0.88181818 0.88636364 0.89090909 0.89545455 0.9 0.90454545 0.90909091 0.91363636 0.91818182 0.92272727 0.92727273 0.93181818 0.93636364 0.94090909 0.94545455 0.95 0.95454545 0.95909091 0.96363636 0.96818182 0.97272727 0.97727273 0.98181818 0.98636364 0.99090909 0.99545455 1 1 1 1 1 1
  point P0 (320, -30)
  point P1 (300, -30)
  point P2 (293.5136, -40)
  point P3 (285.1598, -64.2466)
  point P4 (280, -90)
  point P5 (273.0931, -114.3699)
  point P6 (270, -140)
  point P7 (260, -160)
  point P8 (240, -170)
  point P9 (220, -170)
  point P10 (220, -150)
  point P11 (220, -120)
  point P12 (220, -100)
  point P13 (222.5057, -74.4569)
  point P14 (225.7544, -55.8927)
  point P15 (227.1467, -44.7542)
  point P16 (230, -30)
  point P17 (240, -30)
  point P18 (250, -50)
  point P19 (240, -80)
  point P20 (240, -110)
  point P21 (240, -130)
  point P22 (250, -130)
  point P23 (260, -110)
  point P24 (260, -80)
  point P25 (270, -50)
  point P26 (280, -30)
  point P27 (290, -10)
  point P28 (320, -10)
  point P29 (340, -20)
  point P30 (345.4933, -40)
  point P31 (340, -50)
  point P32 (330, -50)
  point P33 (194.1953, -92.557)
  point P34 (174.703, -108.8006)
  point P35 (160, -110)
  point P36 (150, -100)
  point P37 (140, -80)
  point P38 (140, -90)
  point P39 (140, -110)
  point P40 (135.7182, -108.8006)
  point P41 (130, -100)
  point P42 (130, -80)
  point P43 (130, -70)
  point P44 (130, -50)
  point P45 (127.8284, -34.544)
  point P46 (125.0438, -27.1183)
  point P47 (114.3694, -22.0131)
  point P48 (105.0873, -28.9747)
  point P49 (100, -30)
  point P50 (96.7335, -26.6542)
  point P51 (100, -20)
  point P52 (110, -10)
  point P53 (120, -10)
  point P54 (132.4695, -15.5157)
  point P55 (140, -20)
  point P56 (140, -30)
  point P57 (140, -40)
  point P58 (145.4644, -27.5824)
  point P59 (145.4644, -15.9798)
  point P60 (170, -10)
  point P61 (180, -10)
  point P62 (200, -30)
  point P63 (204.4056, -40)
  point P64 (204.8697, -56.821)
  point P65 (180, -80)
  point P66 (158.9234, -85.5954)
  point P67 (150, -80)
  point P68 (155.6747, -51.7158)
  point P69 (161.2439, -34.544)
  point P70 (180, -34.544)
  point P71 (184.4491, -51.2517)
  point P72 (180, -56.821)
  point P73 (55.0801, -80)
  point P74 (54.6306, -61.3331)
  point P75 (50, -40)
  point P76 (46.0918, -14.1445)
  point P77 (16.8797, -5.6056)
  point P78 (-10, -10)
  point P79 (-15.0288, -31.6717)
  point P80 (-20.4218, -56.821)
  point P81 (-17.2758, -94.1404)
  point P82 (-18.1747, -110.3194)
  point P83 (-25.8147, -74.8156)
  point P84 (-24.4665, -51.2517)
  point P85 (-24.4665, -32.1211)
  point P86 (-30, -20)
  point P87 (-30, -10)
  point P88 (-40, 0)
  point P89 (-51.4314, -4.7067)
  point P90 (-44.2408, -15.0433)
  point P91 (-38.3984, -33.9187)
  point P92 (-39.2972, -51.2517)
  point P93 (-41.0949, -75.265)
  point P94 (-36.1513, -94.1404)
  point P95 (-33.4548, -102.6793)
  point P96 (-27.163, -115.263)
  point P97 (-23.5677, -123.3525)
  point P98 (-16.377, -122.0042)
  point P99 (-5.591, -122.903)
  point P100 (-2.4451, -110.3194)
  point P101 (-10, -100)
  point P102 (0, -70)
  point P103 (3.3973, -43.3565)
  point P104 (10, -30)
  point P105 (30.3622, -51.2517)
  point P106 (30, -70)
  point P107 (35.7552, -90.5451)
  point P108 (35.7552, -104.9264)
  point P109 (40, -120)
  point P110 (46.9906, -125.5995)
  point P111 (54.6306, -117.9595)
  point P112 (40, -160)
  point P113 (34.8564, -172.7882)
  point P114 (20, -170)
  point P115 (-4.6922, -169.1928)
  point P116 (-10.5346, -174.5858)
  point P117 (-10, -160)
  point P118 (-6.9393, -154.8115)
  point P119 (10, -140)
  point P120 (14.1832, -145.8232)
  point P121 (29.4634, -150.3174)
  point P122 (-80, -180)
  point P123 (-90, -180)
  point P124 (-95.5848, -167.2418)
  point P125 (-100, -140)
  point P126 (-110, -170)
  point P127 (-132.6085, -185.7537)
  point P128 (-150, -190)
  point P129 (-170, -180)
  point P130 (-180, -180)
  point P131 (-180, -170)
  point P132 (-180, -160)
  point P133 (-170, -150)
  point P134 (-160, -170)
  point P135 (-145.1313, -164.5195)
  point P136 (-138.8572, -155.9618)
  point P137 (-130, -150)
  point P138 (-120.1495, -136.1316)
  point P139 (-105.9297, -124.2289)
  point P140 (-98.4486, -113.3082)
  point P141 (-128.7551, -114.0565)
  point P142 (-140, -120)
  point P143 (-150, -110)
  point P144 (-150, -90)
  point P145 (-160, -70)
  point P146 (-180, -70)
  point P147 (-190, -60)
  point P148 (-190, -50)
  point P149 (-170, -50)
  point P150 (-145.1313, -48.548)
  point P151 (-130, -50)
  point P152 (-130, -70)
  point P153 (-110.0474, -94.2264)
  point P154 (-92.4621, -95.3488)
  point P155 (-90, -80)
  point P156 (-93.9587, -53.0694)
  point P157 (-90, -40)
  point P158 (-74.5027, -41.0965)
  point P159 (-70, -70)
  point P160 (-70, -90)
  point P161 (-70, -116.0619)
  point P162 (-70, -140)
  point P163 (-70, -154.7191)
  point P164 (-67.3938, -172.7987)
sketch "Sketch43" plane through (0, 0, 0) normal (0, 1, 0) x (1, 0, 0)
  line L0 (264.4869, -130.3819) -> (134.4869, -130.3819)
  line L1 (134.4869, -130.3819) -> (134.4869, -40.3819)
  line L2 (134.4869, -40.3819) -> (264.4869, -40.3819)
  line L3 (264.4869, -40.3819) -> (264.4869, -130.3819)
  dimension "d231" = 130
  dimension "d232" = 90
  constraint horizontal L0
  constraint vertical L1
  constraint horizontal L2
  constraint vertical L3
  measures "d231" distance of L0.start L0.end
  measures "d232" distance of L0.end L1.end
extrude "Extrude18" add sketch "Sketch43" along normal blind 25 separate body makes body 14
ref_plane "WorkPlane21" through (199.4869, 25, 85.3819) normal (0, 1, 0) x (0, 0, 1)
sketch "Sketch44" plane through (199.4869, 25, 85.3819) normal (0, 1, 0) x (1, 0, 0)
  line L0 (65, -45) -> (-65, 45) construction
  line L1 (-15, 25.9808) -> (-30, 0)
  line L2 (-30, 0) -> (-15, -25.9808)
  line L3 (-15, -25.9808) -> (15, -25.9808)
  line L4 (15, -25.9808) -> (30, 0)
  line L5 (30, 0) -> (15, 25.9808)
  line L6 (15, 25.9808) -> (-15, 25.9808)
  dimension "d236" = 60
  constraint horizontal L6
  measures "d236" distance of L2.end L5.end
extrude "Extrude19" add sketch "Sketch44" along normal blind 75 bodies 14
ref_plane "WorkPlane22" through (199.4869, 100, 85.3819) normal (0, 1, 0) x (0, 0, 1)
sketch "Sketch45" plane through (199.4869, 100, 85.3819) normal (0, 1, 0) x (1, 0, 0)
  circle A0 centre (0, 0) radius 45
  constraint coincident A0.centre origin
extrude "Extrude20" add sketch "Sketch45" along normal blind 20 bodies 14
sketch "Sketch46" plane through (0, 120, 0) normal (0, 1, 0) x (-1, 0, 0)
  circle A0 centre (-199.4869, 85.3819) radius 45
  line L0 (-199.4869, 85.3819) -> (-199.4869, 40.3819) construction
  line L1 (-209.4869, 41.5071) -> (-209.4869, 129.2567)
  line L2 (-189.4869, 41.5071) -> (-189.4869, 129.2567)
  dimension "d242" = 20
  constraint coincident A0.centre L0.start
  constraint coincident A0 L0.end
  constraint vertical L0
  constraint coincident A0 L1.start
  constraint coincident A0 L1.end
  constraint vertical L1
  constraint symmetric L0 L1.start L2.start
  constraint symmetric L0 L1.end L2.end
  measures "d242" distance of L1 L2
extrude "Extrude21" cut sketch "Sketch46" against normal blind 10 contours A0 L1 L2 bodies 14
sketch "Sketch47" plane through (0, 120, 0) normal (0, 1, 0) x (-1, 0, 0)
  line L0 (-209.4869, 41.5071) -> (-209.4869, 129.2567)
  arc A0 (-209.4869, 129.2567) -> (-209.4869, 41.5071) centre (-199.4869, 85.3819) ccw
  circle A1 centre (-199.4869, 85.3819) radius 20 construction
  line L1 (-199.4869, 65.3819) -> (-219.4869, 85.3819)
  line L2 (-219.4869, 85.3819) -> (-199.4869, 105.3819)
  line L3 (-199.4869, 105.3819) -> (-179.4869, 85.3819)
  line L4 (-179.4869, 85.3819) -> (-199.4869, 65.3819)
  line L5 (-199.4869, 65.3819) -> (-199.4869, 105.3819) construction
  line L6 (-219.4869, 85.3819) -> (-179.4869, 85.3819) construction
  point P0 (-199.4869, 85.3819)
  dimension "d245" = 40
  constraint concentric A0 A1
  constraint coincident A1 L1.start
  constraint coincident L5 P0
  constraint coincident L6 P0
  constraint coincident P0 A0.centre
  constraint equal L2 L4
  constraint equal L1 L3
  constraint vertical L5
  constraint coincident A1 L1.end
  constraint horizontal L6
  measures "d245" diameter of A1
extrude "Extrude22" cut sketch "Sketch47" against normal up to surface (120 mm away) contours L0 L1 L2 | L0 L1 L2 L3 L4 bodies 14